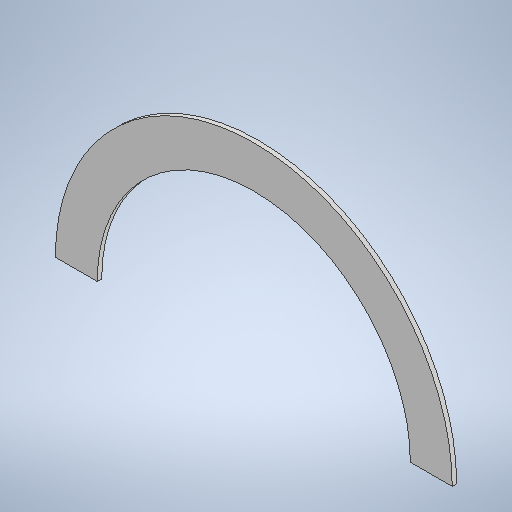
# Autodesk Inventor part: Кольцо заглушки ревиз. окна фильтра D1200
Saved by Autodesk Inventor 2025 (Build 290162010, 162A)
## iProperties
Created: 2025-02-12
Part Number: Кольцо заглушки ревиз. окна фильтра D1200
Material: Generic
Document SubType Name: Sheet Metal
Designer: pokla
Density: 1 g/cm^3
Flat Pattern Width: 27 cm
Flat Pattern Length: 54 cm
Flat Pattern Area: 1458 cm^2
Sheet Metal Rule: Default_mm
Sheet Metal Width: 270,000 mm
Sheet Metal Length: 540,000 mm
Sheet Metal Area: 145800,000 mm^2
Appearance: Default
Author: pokla
Autodesk Inventor part; units mm, degrees
ref_plane "YZ Plane" through (0, 0, 0) normal (1, 0, 0) x (0, 1, 0)
ref_plane "XZ Plane" through (0, 0, 0) normal (0, 1, 0) x (-1, 0, 0)
ref_plane "XY Plane" through (0, 0, 0) normal (0, 0, 1) x (1, 0, 0)
sketch "Sketch1" plane through (0, 0, 0) normal (0, 1, 0) x (-1, 0, 0)
  circle A0 centre (0, 0) radius 213
  circle A1 centre (0, 0) radius 270
  line L0 (270, 0) -> (213, 0)
  line L1 (-213, 0) -> (-270, 0)
  point P0 (241.5, 0)
  point P1 (-241.5, 0)
  dimension "d0" = 426
  dimension "d1" = 540
  constraints: 4 end point, 4 point on circle, 2 centre point, 2 coincident, 2 horizontal, 2 horizontal alignment, 2 midpoint
  measures "d0" diameter of A0
  measures "d1" diameter of A1
extrude "Extrusion1" add sketch "Sketch1" along normal blind 6 contours A0 L1 A1 L0 picked at (-3.3783, 250.7574)
equation "\"d1\" = Внеш_диам_заглушки_ревиз_окна"
equation "\"BendRadius\" = Thickness"
equation "\"BendReliefWidth\" = Thickness"
equation "\"BendReliefDepth\" = 0.5 * Thickness"
equation "\"CornerReliefSize\" = 4 * Thickness"
equation "\"MinimumRemnant\" = 2 * Thickness"
equation "\"TransitionRadius\" = BendRadius"
equation "\"JacobiRadiusSize\" = BendRadius"
equation "\"GapSize\" = Thickness"
equation "\"Внеш_диам_заглушки_ревиз_окна\" = 540"
equation "\"Thickness\" = 6"
body "Solid1"
